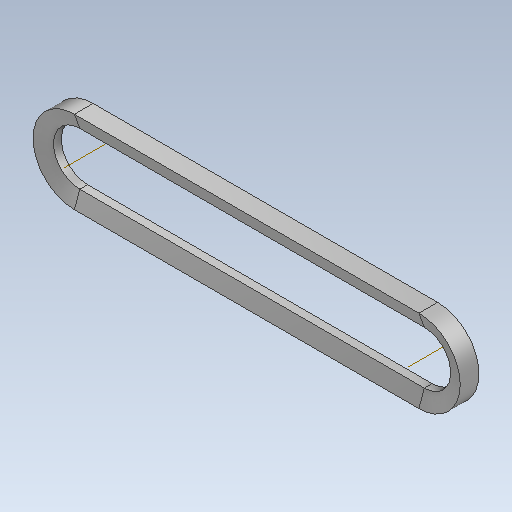
# Autodesk Inventor part: V-Belt
Saved by Autodesk Inventor 2021.1 (Build 251245000, 245)
## iProperties
Created: 2021-01-01
Part Number: V-Belt
Material: Rubber
Document SubType Name: Modeling
Designer: Bolisteward
Density: 0.93 g/cm^3
Appearance: Rubber - Black - Version 1.1
CustomPartVersion: 1
Author: Bolisteward
Autodesk Inventor part; units mm, degrees
ref_plane "YZ Plane" through (0, 0, 0) normal (1, 0, 0) x (0, 1, 0)
ref_plane "XZ Plane" through (0, 0, 0) normal (0, 1, 0) x (-1, 0, 0)
sketch "Sketch Path" plane through (0, 0, 0) normal (0, 0, 1) x (1, 0, 0)
  arc A0 (0, -20) -> (0, 20) centre (0, 0) ccw
  arc A1 (-184, 20) -> (-184, -20) centre (-184, 0) ccw
  line L0 (-184, 20) -> (0, 20)
  line L1 (0, -20) -> (-184, -20)
  constraints: 4 end point, 4 point on circle, 2 centre point
ref_plane "Cross Section Plane" through (0, 20, 0) normal (-1, 0, 0) x (0, 0, 1)
sketch "Cross Section" plane through (0, 20, 0) normal (-1, 0, 0) x (0, 0, 1)
  line L0 (0, 2.069) -> (0, -5.931) construction
  line L1 (-4.25, 0) -> (4.25, 0) construction
  line L2 (-5.0031, 2.069) -> (5.0031, 2.069)
  line L3 (5.0031, 2.069) -> (2.0913, -5.931)
  line L4 (2.0913, -5.931) -> (-2.0913, -5.931)
  line L5 (-2.0913, -5.931) -> (-5.0031, 2.069)
  point P0 (0, 0)
  point P1 (0, 0)
  point P2 (0, 0)
  dimension "d0" = 8.5
  dimension "d1" = 2.069
  dimension "d2" = 40
  dimension "d3" = 8
  constraints: 12 end point, 3 midpoint, 2 parallel, 2 point on line, 1 coincident, 1 perpendicular, 1 vertical, 1 other
  measures "d0" distance of L1.start L1.end
  measures "d1" distance between parallel lines of L2 L1
  measures "d2" angle of L5 L3
  measures "d3" distance between parallel lines of L4 L2
sweep "Belt" add profiles "Cross Section" path "Sketch Path"
equation "\"d0\" = da_Bw"
equation "\"d1\" = da_Hw"
equation "\"d2\" = da_Alfa"
equation "\"d3\" = da_H"
equation "\"da_Alfa\" = 40deg"
equation "\"da_H\" = 8"
equation "\"da_Bw\" = 8.5"
equation "\"da_Hw\" = 2.06901"
body "Solid1"
